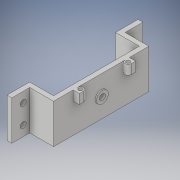
# Autodesk Inventor part: yaxis_clamp1
Saved by Autodesk Inventor 2019 (Build 230136000, 136)
## iProperties
Created: 2020-02-02
Material: Generic
Document SubType Name: Modeling
Designer: Nishant
Density: 1 g/cm^3
Appearance: Default
Author: Nishant
Autodesk Inventor part; units mm, degrees
ref_plane "YZ Plane" through (0, 0, 0) normal (1, 0, 0) x (0, 1, 0)
ref_plane "XZ Plane" through (0, 0, 0) normal (0, 1, 0) x (-1, 0, 0)
ref_plane "XY Plane" through (0, 0, 0) normal (0, 0, 1) x (1, 0, 0)
sketch "Sketch1" plane through (0, 0, 0) normal (1, 0, 0) x (0, 1, 0)
  line L0 (0, 0) -> (33, 0)
  line L1 (33, 0) -> (33, 19)
  line L2 (33, 19) -> (0, 19)
  line L3 (0, 19) -> (0, 0)
  circle A0 centre (24.5, 9.5) radius 2.5
  circle A1 centre (8.5, 9.5) radius 2.5
  dimension "d0" = 33
  dimension "d1" = 19
  dimension "d2" = 33
  dimension "d3" = 19
  dimension "d6" = 5
  dimension "d8" = 5
  constraints: 8 end point, 2 centre point, 1 horizontal, 1 perpendicular, 1 vertical
  measures "d0" distance of L0.start L0.end
  measures "d1" distance of L0.end L1.end
  measures "d2" distance of L1.end L2.end
  measures "d3" distance of L2.end L0.start
  measures "d6" diameter of A0
  measures "d8" diameter of A1
extrude "Extrusion1" add sketch "Sketch1" along normal blind 4
sketch "Sketch2" plane through (0, 33, 19) normal (0, 1, 0) x (1, 0, 0)
  line L0 (0, 19) -> (4, 19) projected
  line L1 (0, 19) -> (24, 19)
  line L2 (24, 19) -> (24, 15)
  line L3 (24, 15) -> (0, 15)
  line L4 (0, 19) -> (0, 0) projected
  line L5 (0, 15) -> (0, 19)
  dimension "d11" = 24
  dimension "d12" = 4
  dimension "d13" = 24
  constraints: 8 end point, 2 perpendicular, 1 collinear
  measures "d11" distance of L0.start L1.end
  measures "d12" distance of L1.end L2.end
  measures "d13" distance of L2.end L3.end
extrude "Extrusion2" add sketch "Sketch2" against normal blind 33
sketch "Sketch3" plane through (0, 33, 19) normal (0, 1, 0) x (1, 0, 0)
  line L0 (4, 15) -> (24, 15) projected
  line L1 (24, 15) -> (24, 95)
  line L2 (24, 15) -> (20, 15)
  line L3 (20, 15) -> (20, 95)
  line L4 (20, 95) -> (24, 95)
  point P0 (0, 19)
  dimension "d16" = 80
  dimension "d17" = 4
  dimension "d18" = 80
  dimension "d19" = 4
  constraints: 8 end point, 1 perpendicular, 1 point on line, 1 vertical
  measures "d16" distance of L0.end L1.end
  measures "d17" distance of L0.end L2.end
  measures "d18" distance of L2.end L3.end
  measures "d19" distance of L3.end L1.end
extrude "Extrusion3" add sketch "Sketch3" against normal blind 33
sketch "Sketch4" plane through (0, 33, 19) normal (0, 1, 0) x (1, 0, 0)
  line L0 (24, 95) -> (20, 95) projected
  line L1 (24, 95) -> (0, 95)
  line L2 (0, 95) -> (0, 91)
  line L3 (0, 91) -> (24, 91)
  line L4 (24, 15) -> (24, 95) projected
  line L5 (24, 91) -> (24, 95)
  point P0 (0, 19)
  dimension "d22" = 24
  dimension "d23" = 4
  dimension "d24" = 24
  dimension "d25" = 4
  constraints: 8 end point, 2 perpendicular, 1 collinear, 1 point on line
  measures "d22" distance of L0.start L1.end
  measures "d23" distance of L1.end L2.end
  measures "d24" distance of L2.end L3.end
  measures "d25" distance of L3.end L0.start
extrude "Extrusion4" add sketch "Sketch4" against normal blind 33
sketch "Sketch5" plane through (0, 33, 19) normal (0, 1, 0) x (1, 0, 0)
  line L0 (0, 91) -> (0, 110)
  line L1 (0, 110) -> (4, 110)
  line L2 (4, 110) -> (4, 91)
  line L3 (20, 91) -> (0, 91) projected
  line L4 (4, 91) -> (0, 91)
  point P0 (0, 19)
  dimension "d28" = 19
  dimension "d29" = 4
  dimension "d30" = 19
  dimension "d31" = 4
  constraints: 8 end point, 2 perpendicular, 1 vertical
  measures "d28" distance of L0.start L0.end
  measures "d29" distance of L0.end L1.end
  measures "d30" distance of L1.end L2.end
  measures "d31" distance of L2.end L0.start
extrude "Extrusion5" add sketch "Sketch5" against normal blind 33
sketch "Sketch6" plane through (4, 33, -76) normal (1, 0, 0) x (0, 0, -1)
  line L0 (15, 0) -> (-4, 0) projected
  circle A0 centre (5.5, -8.5) radius 2.5
  circle A1 centre (5.5, -24.5) radius 2.5
  point P0 (-76, -33)
  dimension "d36" = 5
  dimension "d38" = 5
  constraints: 2 centre point
  measures "d36" diameter of A0
  measures "d38" diameter of A1
hole "Hole1" at (4, 24.5, -81.5) at (4, 8.5, -81.5) direction (-1, 0, 0) diameter 5 end through all both
sketch "Sketch7" plane through (24, 0, 4) normal (1, 0, 0) x (0, 0, -1)
  line L0 (0, 33) -> (80, 33) projected
  circle A0 centre (40, 16.5) radius 5
  circle A1 centre (40, 16.5) radius 2.5
  point P0 (4, 0)
  point P1 (0, 0)
  dimension "d46" = 10
  dimension "d47" = 5
  constraints: 2 centre point, 1 coincident
  measures "d46" diameter of A0
  measures "d47" diameter of A1
hole "Hole2" at (24, 16.5, -36) direction (-1, 0, 0) diameter 5 end through all both
extrude "Extrusion6" add sketch "Sketch7" along normal blind 1
sketch "Sketch8" plane through (0, 33, 19) normal (0, 1, 0) x (1, 0, 0)
  line L0 (24, 31.4) -> (29.2, 31.4)
  line L1 (29.2, 31.4) -> (29.2, 35)
  line L2 (26.6, 37.6) -> (26.6, 37.6)
  line L3 (24, 35) -> (24, 31.4)
  arc A0 (26.6, 37.6) -> (24, 35) centre (26.6, 35) ccw
  arc A1 (29.2, 35) -> (26.6, 37.6) centre (26.6, 35) ccw
  circle A2 centre (26.6, 35) radius 1.6
  point P0 (0, 19)
  point P1 (24, 15)
  point P2 (29.2, 37.6)
  point P3 (24, 37.6)
  dimension "d58" = 5.2
  dimension "d59" = 6.2
  dimension "d60" = 5.2
  dimension "d61" = 6.2
  dimension "d62" = 2.6
  dimension "d63" = 3.2
  constraints: 8 end point, 4 point on circle, 4 point on line, 4 tangent, 3 centre point, 2 perpendicular, 1 coincident, 1 concentric
  measures "d58" distance of L0.start L0.end
  measures "d59" distance of L0.end point (29.2, 37.6)
  measures "d60" distance of point (29.2, 37.6) point (24, 37.6)
  measures "d61" distance of point (24, 37.6) L0.start
  measures "d62" radius of A0
  measures "d63" diameter of A2
extrude "Extrusion7" add sketch "Sketch8" against normal blind 8
sketch "Sketch9" plane through (0, 33, 19) normal (0, 1, 0) x (1, 0, 0)
  line L0 (24, 95) -> (4, 95) projected
  line L1 (24, 95) -> (24, 15) projected
  line L2 (24, 78.6) -> (29.2, 78.6)
  line L3 (29.2, 78.6) -> (29.2, 75)
  line L4 (26.6, 72.4) -> (26.6, 72.4)
  line L5 (24, 75) -> (24, 78.6)
  arc A0 (26.6, 72.4) -> (29.2, 75) centre (26.6, 75) ccw
  arc A1 (24, 75) -> (26.6, 72.4) centre (26.6, 75) ccw
  circle A2 centre (26.6, 75) radius 1.6
  point P0 (0, 19)
  point P1 (29.2, 72.4)
  point P2 (24, 72.4)
  dimension "d67" = 5.2
  dimension "d68" = 6.2
  dimension "d69" = 5.2
  dimension "d70" = 6.2
  dimension "d71" = 2.6
  dimension "d72" = 3.2
  constraints: 8 end point, 6 point on line, 4 point on circle, 4 tangent, 3 centre point, 1 coincident, 1 concentric, 1 perpendicular
  measures "d67" distance of L2.start L2.end
  measures "d68" distance of L2.end point (29.2, 72.4)
  measures "d69" distance of point (29.2, 72.4) point (24, 72.4)
  measures "d70" distance of point (24, 72.4) L2.start
  measures "d71" radius of A0
  measures "d72" diameter of A2
extrude "Extrusion8" add sketch "Sketch9" against normal blind 8
body "Solid1"
